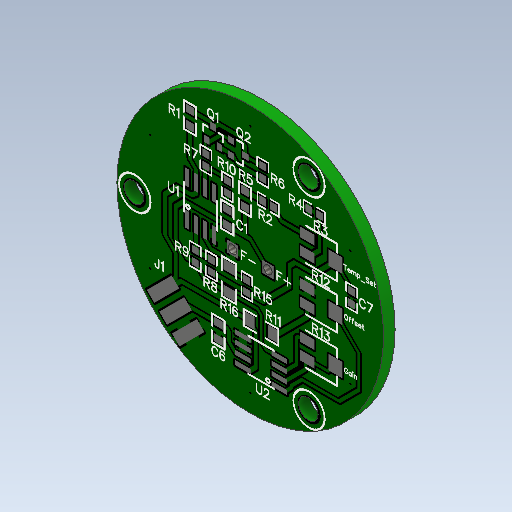
# Autodesk Inventor part: Filament Board
Saved by Autodesk Inventor 2020 (Build 240168000, 168)
## iProperties
Created: 2018-03-05
Part Number: Filament Board
Material: Generic
Document SubType Name: Modeling
Designer: Alex
Density: 1 g/cm^3
Appearance: Default
Author: Alex
Autodesk Inventor part; units mm, degrees
ref_plane "YZ Plane" through (0, 0, 0) normal (1, 0, 0) x (0, 1, 0)
ref_plane "XZ Plane" through (0, 0, 0) normal (0, 1, 0) x (-1, 0, 0)
ref_plane "XY Plane" through (0, 0, 0) normal (0, 0, 1) x (1, 0, 0)
sketch "Sketch1" plane through (0, 0, 0) normal (0, 0, 1) x (1, 0, 0)
  circle A0 centre (0, 0) radius 19.05
  dimension "d0" = 38.1
  constraints: 1 centre point, 1 coincident
  measures "d0" diameter of A0
extrude "Extrusion1" add sketch "Sketch1" along normal blind 1.651
sketch "Sketch2" plane through (0, 0, 1.651) normal (0, 0, 1) x (1, 0, 0)
  circle A0 centre (0, 0) radius 19.05 projected
  line L0 (-19.05, 19.05) -> (19.05, 19.05) construction
  line L1 (19.05, 19.05) -> (19.05, -19.05) construction
  line L2 (19.05, -19.05) -> (-19.05, -19.05) construction
  line L3 (-19.05, -19.05) -> (-19.05, 19.05) construction
  point P0 (0, 19.05)
  point P1 (-19.05, 0)
  point P2 (0, 19.05)
  point P3 (-19.05, 0)
  constraints: 4 point on circle, 2 horizontal alignment, 2 midpoint, 2 vertical alignment, 2 other
decal "Decal1"
sketch "Sketch3" plane through (0, 0, 1.651) normal (0, 0, 1) x (1, 0, 0)
  circle A0 centre (-16.5947, 0) radius 1.397
  line L0 (19.05, -19.05) -> (-19.05, -19.05) construction
  line L1 (-19.05, -19.05) -> (-19.05, 19.05) construction
  line L2 (-19.05, 19.05) -> (19.05, 19.05) construction
  line L3 (19.05, 19.05) -> (19.05, -19.05) construction
  line L4 (19.05, -19.05) -> (-19.05, 19.05) construction
  line L5 (-19.05, -19.05) -> (19.05, 19.05) construction
  circle A1 centre (8.2973, 14.3714) radius 1.397
  circle A2 centre (8.2973, -14.3714) radius 1.397
  line L6 (-16.5947, 0) -> (8.2973, 14.3714) construction
  line L7 (8.2973, 14.3714) -> (8.2973, -14.3714) construction
  line L8 (8.2973, -14.3714) -> (-16.5947, 0) construction
  circle A3 centre (-2.54, 0) radius 0.6096
  circle A4 centre (2.54, 0) radius 0.6096
  point P0 (0, 0)
  point P1 (0, 0)
  dimension "d8" = 2.794
  dimension "d9" = 38.1
  dimension "d11" = 19.05
  dimension "d13" = 1.2192
  dimension "d14" = 5.08
  dimension "d15" = 2.54
  dimension "d25" = 24.892
  dimension "d26" = 2.4553
  constraints: 18 end point, 5 centre point, 4 coincident, 3 equal radius, 2 horizontal alignment, 2 midpoint, 2 parallel, 2 perpendicular, 1 horizontal, 7 other
  measures "d8" diameter of A0
  measures "d9" distance of L1.end L2.end
  measures "d11" distance from line of L6.start L2
  measures "d13" diameter of A3
  measures "d14" distance of A4.centre A3.centre
  measures "d15" distance of A3.centre point (0, 0)
  measures "d25" distance from line of L7 L6.start
  measures "d26" distance from line of L1 L6.start
extrude "Extrusion2" cut sketch "Sketch3" against normal through all
sketch "Sketch5" plane through (0, 0, 0) normal (0, 0, -1) x (-1, 0, 0)
  circle A0 centre (0, 0) radius 19.05 projected
  line L0 (-19.05, 19.05) -> (19.05, 19.05) construction
  line L1 (19.05, 19.05) -> (19.05, -19.05) construction
  line L2 (19.05, -19.05) -> (-19.05, -19.05) construction
  line L3 (-19.05, -19.05) -> (-19.05, 19.05) construction
  point P0 (-19.05, 0)
  point P1 (0, 19.05)
  point P2 (0, 19.05)
  point P3 (-19.05, 0)
  constraints: 3 point on circle, 2 horizontal alignment, 2 midpoint, 2 vertical alignment, 1 horizontal, 2 other
decal "Decal3"
body "Solid1"
